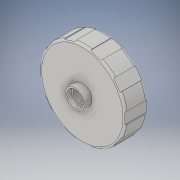
# Autodesk Inventor part: Bauteil1
Saved by Autodesk Inventor 2019 (Build 230136000, 136)
## iProperties
Created: 2024-05-17
Part Number: Bauteil1
Material: Generisch
Document SubType Name: Modeling
Designer: nic
Density: 1 g/cm^3
Appearance: Vorgabe
Author: nic
Autodesk Inventor part; units mm, degrees
ref_plane "YZ Plane" through (0, 0, 0) normal (1, 0, 0) x (0, 1, 0)
ref_plane "XZ Plane" through (0, 0, 0) normal (0, 1, 0) x (-1, 0, 0)
ref_plane "XY Plane" through (0, 0, 0) normal (0, 0, 1) x (1, 0, 0)
sketch "Skizze1" plane through (0, 0, 0) normal (0, 0, 1) x (1, 0, 0)
  circle A0 centre (0, 0) radius 77
  circle A1 centre (0, 0) radius 11.415
  dimension "d0" = 154
  dimension "d1" = 22.83
  constraints: 2 centre point, 2 coincident
  measures "d0" diameter of A0
  measures "d1" diameter of A1
extrude "Extrusion1" add sketch "Skizze1" along normal blind 40.6
sketch "Skizze2" plane through (0, 0, 0) normal (0, 0, -1) x (-1, 0, 0)
  circle A0 centre (0, 0) radius 16.25
  dimension "d4" = 32.5
  constraints: 1 centre point, 1 coincident
  measures "d4" diameter of A0
extrude "Extrusion2" cut sketch "Skizze2" against normal blind 11
sketch "Skizze3" plane through (0, 0, 11) normal (0, 0, -1) x (-1, 0, 0)
  circle A0 centre (0, 0) radius 15
  dimension "d7" = 30
  constraints: 1 centre point, 1 coincident
  measures "d7" diameter of A0
extrude "Extrusion3" cut sketch "Skizze3" against normal blind 8
fillet "Rundung1" radius 2 1 edges at (15, 0, 11)
fillet "Rundung2" radius 2 1 edges at (16.25, 0, 0)
fillet "Rundung3" radius 4 2 edges at (-77, 0, 0) (-77, 0, 40.6)
sketch "Skizze4" plane through (0, 0, 40.6) normal (0, 0, 1) x (1, 0, 0)
  circle A0 centre (0, 0) radius 11.415 projected
  circle A1 centre (0, 0) radius 17.415
  dimension "d13" = 6
  constraints: 1 centre point
  measures "d13" radial gap between concentric circles of A0 A1
extrude "Extrusion4" add sketch "Skizze4" along normal blind 13
sketch "Skizze5" plane through (0, 0, 53.6) normal (0, 0, 1) x (1, 0, 0)
  circle A0 centre (0, 0) radius 14.75
  dimension "d16" = 29.5
  constraints: 1 centre point, 1 coincident
  measures "d16" diameter of A0
extrude "Extrusion5" cut sketch "Skizze5" against normal blind 8
sketch "Skizze6" plane through (0, 0, 0) normal (0, 0, -1) x (-1, 0, 0)
  line L0 (-78.4205, -10.1285) -> (-75.313, -10.1285)
  line L1 (-75.313, -10.1285) -> (-75.313, 10.1285)
  line L2 (-75.313, 10.1285) -> (-78.4205, 10.1285)
  line L3 (-78.4205, 10.1285) -> (-78.4205, -10.1285)
  line L4 (-78.4205, -10.1285) -> (-75.313, 10.1285) construction
  line L5 (-75.313, -10.1285) -> (-78.4205, 10.1285) construction
  line L6 (-57.4901, -54.2886) -> (-54.9761, -52.462)
  line L7 (-54.9761, -52.462) -> (-66.8829, -36.0737)
  line L8 (-66.8829, -36.0737) -> (-69.3969, -37.9002)
  line L9 (-69.3969, -37.9002) -> (-57.4901, -54.2886)
  line L10 (-57.4901, -54.2886) -> (-66.8829, -36.0737) construction
  line L11 (-54.9761, -52.462) -> (-69.3969, -37.9002) construction
  line L12 (-14.6004, -77.7122) -> (-13.6402, -74.7568)
  line L13 (-13.6402, -74.7568) -> (-32.9058, -68.497)
  line L14 (-32.9058, -68.497) -> (-33.8661, -71.4524)
  line L15 (-33.8661, -71.4524) -> (-14.6004, -77.7122)
  line L16 (-14.6004, -77.7122) -> (-32.9058, -68.497) construction
  line L17 (-13.6402, -74.7568) -> (-33.8661, -71.4524) construction
  line L18 (33.8661, -71.4524) -> (32.9058, -68.497)
  line L19 (32.9058, -68.497) -> (13.6402, -74.7568)
  line L20 (13.6402, -74.7568) -> (14.6004, -77.7122)
  line L21 (14.6004, -77.7122) -> (33.8661, -71.4524)
  line L22 (33.8661, -71.4524) -> (13.6402, -74.7568) construction
  line L23 (32.9058, -68.497) -> (14.6004, -77.7122) construction
  line L24 (69.3969, -37.9002) -> (66.8829, -36.0737)
  line L25 (66.8829, -36.0737) -> (54.9761, -52.462)
  line L26 (54.9761, -52.462) -> (57.4901, -54.2886)
  line L27 (57.4901, -54.2886) -> (69.3969, -37.9002)
  line L28 (69.3969, -37.9002) -> (54.9761, -52.462) construction
  line L29 (66.8829, -36.0737) -> (57.4901, -54.2886) construction
  line L30 (78.4205, 10.1285) -> (75.313, 10.1285)
  line L31 (75.313, 10.1285) -> (75.313, -10.1285)
  line L32 (75.313, -10.1285) -> (78.4205, -10.1285)
  line L33 (78.4205, -10.1285) -> (78.4205, 10.1285)
  line L34 (78.4205, 10.1285) -> (75.313, -10.1285) construction
  line L35 (75.313, 10.1285) -> (78.4205, -10.1285) construction
  line L36 (57.4901, 54.2886) -> (54.9761, 52.462)
  line L37 (54.9761, 52.462) -> (66.8829, 36.0737)
  line L38 (66.8829, 36.0737) -> (69.3969, 37.9002)
  line L39 (69.3969, 37.9002) -> (57.4901, 54.2886)
  line L40 (57.4901, 54.2886) -> (66.8829, 36.0737) construction
  line L41 (54.9761, 52.462) -> (69.3969, 37.9002) construction
  line L42 (14.6004, 77.7122) -> (13.6402, 74.7568)
  line L43 (13.6402, 74.7568) -> (32.9058, 68.497)
  line L44 (32.9058, 68.497) -> (33.8661, 71.4524)
  line L45 (33.8661, 71.4524) -> (14.6004, 77.7122)
  line L46 (14.6004, 77.7122) -> (32.9058, 68.497) construction
  line L47 (13.6402, 74.7568) -> (33.8661, 71.4524) construction
  line L48 (-33.8661, 71.4524) -> (-32.9058, 68.497)
  line L49 (-32.9058, 68.497) -> (-13.6402, 74.7568)
  line L50 (-13.6402, 74.7568) -> (-14.6004, 77.7122)
  line L51 (-14.6004, 77.7122) -> (-33.8661, 71.4524)
  line L52 (-33.8661, 71.4524) -> (-13.6402, 74.7568) construction
  line L53 (-32.9058, 68.497) -> (-14.6004, 77.7122) construction
  line L54 (-69.3969, 37.9002) -> (-66.8829, 36.0737)
  line L55 (-66.8829, 36.0737) -> (-54.9761, 52.462)
  line L56 (-54.9761, 52.462) -> (-57.4901, 54.2886)
  line L57 (-57.4901, 54.2886) -> (-69.3969, 37.9002)
  line L58 (-69.3969, 37.9002) -> (-54.9761, 52.462) construction
  line L59 (-66.8829, 36.0737) -> (-57.4901, 54.2886) construction
  point P0 (0, 0)
  point P1 (-76.8667, 0)
  point P2 (-62.1865, -45.1811)
  point P3 (-23.7531, -73.1046)
  point P4 (23.7531, -73.1046)
  point P5 (62.1865, -45.1811)
  point P6 (76.8667, 0)
  point P7 (62.1865, 45.1811)
  point P8 (23.7531, 73.1046)
  point P9 (-23.7531, 73.1046)
  point P10 (-62.1865, 45.1811)
  dimension "d21" = 360
  constraints: 120 end point, 20 midpoint, 2 parallel, 1 horizontal, 1 perpendicular, 111 other
extrude "Extrusion6" cut sketch "Skizze6" against normal through all
